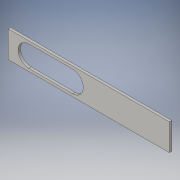
# Autodesk Inventor part: front
Saved by Autodesk Inventor 2016 (Build 200138000, 138)
## iProperties
Created: 2017-09-18
Part Number: front
Material: Generic
Document SubType Name: Modeling
Designer: Student
Density: 1 g/cm^3
Appearance: Default
Author: Student
Autodesk Inventor part; units mm, degrees
ref_plane "YZ Plane" through (0, 0, 0) normal (1, 0, 0) x (0, 1, 0)
ref_plane "XZ Plane" through (0, 0, 0) normal (0, 1, 0) x (-1, 0, 0)
ref_plane "XY Plane" through (0, 0, 0) normal (0, 0, 1) x (1, 0, 0)
sketch "Sketch1" plane through (0, 0, 0) normal (0, 0, 1) x (1, 0, 0)
  line L0 (-268.1444, 21.3208) -> (39.7036, 21.3208)
  line L1 (39.7036, 21.3208) -> (39.7036, -29.4792)
  line L2 (39.7036, -29.4792) -> (-268.1444, -29.4792)
  line L3 (-268.1444, -29.4792) -> (-268.1444, 21.3208)
  point P0 (0, 0)
  dimension "d0" = 50.8
  dimension "d1" = 307.848
  constraints: 8 end point, 2 parallel, 1 horizontal, 1 perpendicular
  measures "d0" distance of L0.end L1.end
  measures "d1" distance of L0.start L0.end
extrude "Extrusion1" add sketch "Sketch1" along normal blind 4.699
sketch "Sketch3" plane through (0, 0, 4.699) normal (0, 0, 1) x (1, 0, 0)
  line L0 (-228.8776, -4.0792) -> (-144.9306, -4.0792) construction
  line L1 (-228.8776, -24.3992) -> (-144.9306, -24.3992)
  line L2 (-144.9306, 16.2408) -> (-228.8776, 16.2408)
  arc A0 (-228.8776, 16.2408) -> (-228.8776, -24.3992) centre (-228.8776, -4.0792) ccw
  arc A1 (-144.9306, -24.3992) -> (-144.9306, 16.2408) centre (-144.9306, -4.0792) ccw
  line L3 (-268.1444, 21.3208) -> (-268.1444, -29.4792) projected
  point P0 (0, 0)
  point P1 (-186.9041, -4.0792)
  point P2 (-249.1976, -4.0792)
  point P3 (-268.1444, -4.0792)
  point P4 (-268.1444, -4.0792)
  dimension "d4" = 83.947
  dimension "d5" = 40.64
  constraints: 8 end point, 5 point on circle, 4 tangent, 3 midpoint, 2 centre point, 1 horizontal, 1 parallel
  measures "d4" distance of L0.start L0.end
  measures "d5" diameter of A1
extrude "Extrusion2" cut sketch "Sketch3" against normal blind 25.4
body "Solid1"
